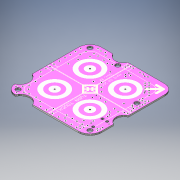
# Autodesk Inventor part: Eagle PCB rev 38
Saved by Autodesk Inventor 2016 (Build 200138000, 138)
## iProperties
Created: 2017-04-10
Part Number: Eagle PCB rev 38
Material: Generic
Document SubType Name: Modeling
Designer: Samuel Clay
Density: 1 g/cm^3
Appearance: Default
Author: Samuel Clay
Autodesk Inventor part; units mm, degrees
(part 1 of 3)
ref_plane "YZ Plane" through (0, 0, 0) normal (1, 0, 0) x (0, 1, 0)
ref_plane "XZ Plane" through (0, 0, 0) normal (0, 1, 0) x (-1, 0, 0)
ref_plane "XY Plane" through (0, 0, 0) normal (0, 0, 1) x (1, 0, 0)
sketch "PCB" plane through (0, 0, 0) normal (0, 0, 1) x (1, 0, 0)
  line L0 (18.4531, -13.3626) -> (18.4531, -8.3763)
  line L1 (17.4012, -16.4615) -> (17.5952, -16.1907)
  line L2 (4.9153, 16.5103) -> (4.4111, 16.3752)
  line L3 (13.6552, 10.6901) -> (13.633, 10.7727)
  line L4 (17.0691, 7.2094) -> (17.0086, 7.2699)
  line L5 (11.5809, 14.546) -> (11.4982, 14.5239)
  line L6 (14.6575, 2.3946) -> (14.6356, 2.4765)
  line L7 (2.2015, 12.8535) -> (2.1794, 12.9362)
  line L8 (2.1698, 12.7683) -> (2.1583, 12.8112)
  line L9 (-16.4524, -8.5544) -> (-16.6541, -8.2122)
  line L10 (2.0984, 12.8711) -> (2.0165, 12.8931)
  line L11 (-16.2848, -8.9145) -> (-16.4524, -8.5544)
  line L12 (2.1583, 12.8112) -> (2.0984, 12.8711)
  line L13 (-16.1527, -9.2892) -> (-16.2848, -8.9145)
  line L14 (2.1189, 12.9967) -> (2.0362, 13.0189)
  line L15 (-16.0575, -9.6748) -> (-16.1527, -9.2892)
  line L16 (-16, -10.0678) -> (-16.0575, -9.6748)
  line L17 (2.0362, 13.0189) -> (1.9535, 12.9967)
  line L18 (2.0165, 12.8931) -> (1.9347, 12.8711)
  line L19 (17.4509, -10.6455) -> (17.4731, -10.5628)
  line L20 (-15.9808, -10.4646) -> (-16, -10.0678)
  line L21 (-16, -10.8614) -> (-15.9808, -10.4646)
  line L22 (1.9535, 12.9967) -> (1.893, 12.9362)
  line L23 (1.9347, 12.8711) -> (1.8806, 12.8171)
  line L24 (-16.6541, -8.2122) -> (-16.8879, -7.8911)
  line L25 (2.1794, 12.9362) -> (2.1189, 12.9967)
  line L26 (1.893, 12.9362) -> (1.8709, 12.8535)
  line L27 (-18.4531, 13.3626) -> (-18.4531, -6.6988)
  line L28 (-18.0967, -6.8742) -> (-18.4531, -6.6988)
  line L29 (-17.7589, -7.0832) -> (-18.0967, -6.8742)
  line L30 (-17.4429, -7.3239) -> (-17.7589, -7.0832)
  line L31 (1.893, 12.7709) -> (1.9535, 12.7103)
  line L32 (-17.1517, -7.5941) -> (-17.4429, -7.3239)
  line L33 (-16.8879, -7.8911) -> (-17.1517, -7.5941)
  line L34 (-16.0575, -11.2544) -> (-16, -10.8614)
  line L35 (1.9535, 12.7103) -> (2.0362, 12.6882)
  line L36 (-16.1527, -11.6401) -> (-16.0575, -11.2544)
  line L37 (-16.2848, -12.0147) -> (-16.1527, -11.6401)
  line L38 (-16.4524, -12.3748) -> (-16.2848, -12.0147)
  line L39 (-16.6541, -12.717) -> (-16.4524, -12.3748)
  line L40 (-16.8879, -13.0381) -> (-16.6541, -12.717)
  line L41 (-17.1517, -13.3351) -> (-16.8879, -13.0381)
  line L42 (2.0362, 12.6882) -> (2.1189, 12.7103)
  line L43 (-17.2743, -13.4738) -> (-17.1517, -13.3351)
  line L44 (-17.5873, -13.7121) -> (-17.4429, -13.6053)
  line L45 (-18.0967, -14.055) -> (-17.7589, -13.846)
  line L46 (-17.9218, -13.9191) -> (-17.5873, -13.7121)
  line L47 (-18.4531, -14.2304) -> (-18.2747, -14.0928)
  line L48 (-18.4531, -14.2304) -> (-18.0967, -14.055)
  line L49 (-18.2747, -14.0928) -> (-17.9218, -13.9191)
  line L50 (-18.4528, -14.5799) -> (-18.4354, -14.8417)
  line L51 (-18.4354, -14.8417) -> (-18.4009, -15.1019)
  line L52 (2.1189, 12.7103) -> (2.1698, 12.7683)
  line L53 (-18.4009, -15.1019) -> (-18.3495, -15.3592)
  line L54 (-18.3495, -15.3592) -> (-18.2813, -15.6127)
  line L55 (17.3904, -10.706) -> (17.4509, -10.6455)
  line L56 (-18.2813, -15.6127) -> (-18.1967, -15.8611)
  line L57 (-18.1967, -15.8611) -> (-18.096, -16.1034)
  line L58 (-18.096, -16.1034) -> (-17.9797, -16.3387)
  line L59 (-17.9797, -16.3387) -> (-17.8483, -16.5658)
  line L60 (2.1698, 12.7683) -> (2.2015, 12.8535)
  line L61 (-17.8483, -16.5658) -> (-17.7023, -16.7839)
  line L62 (-17.7023, -16.7839) -> (-17.5423, -16.9919)
  line L63 (-17.5423, -16.9919) -> (-17.3691, -17.1891)
  line L64 (-17.3691, -17.1891) -> (-17.1833, -17.3745)
  line L65 (-17.1833, -17.3745) -> (-16.9858, -17.5473)
  line L66 (-16.9858, -17.5473) -> (-16.7775, -17.7069)
  line L67 (17.3077, -10.7282) -> (17.3904, -10.706)
  line L68 (-16.7775, -17.7069) -> (-16.5591, -17.8524)
  line L69 (-16.5591, -17.8524) -> (-16.3317, -17.9834)
  line L70 (-16.3317, -17.9834) -> (-16.0962, -18.0993)
  line L71 (-16.0962, -18.0993) -> (-15.8537, -18.1995)
  line L72 (-15.8537, -18.1995) -> (-15.6051, -18.2836)
  line L73 (-15.6051, -18.2836) -> (-15.3515, -18.3513)
  line L74 (-15.3515, -18.3513) -> (-15.0941, -18.4022)
  line L75 (-15.0941, -18.4022) -> (-14.8339, -18.4362)
  line L76 (-14.8339, -18.4362) -> (-14.572, -18.4531)
  line L77 (-14.4849, -18.4531) -> (-14.3449, -18.2747)
  line L78 (-14.572, -18.4531) -> (-14.4849, -18.4531)
  line L79 (-14.3095, -18.0967) -> (-14.4849, -18.4531)
  line L80 (-14.1712, -17.9218) -> (-14.3449, -18.2747)
  line L81 (-14.1005, -17.7589) -> (-14.3095, -18.0967)
  line L82 (-13.9642, -17.5873) -> (-14.1712, -17.9218)
  line L83 (-13.8598, -17.4429) -> (-13.9642, -17.5873)
  line L84 (17.2251, -10.706) -> (17.3077, -10.7282)
  line L85 (17.6003, 4.5815) -> (17.5782, 4.6641)
  line L86 (14.3966, -4.3715) -> (14.3361, -4.311)
  line L87 (3.3469, 15.3988) -> (3.3248, 15.4815)
  line L88 (3.3027, 15.2941) -> (3.2926, 15.3318)
  line L89 (17.5782, 4.6641) -> (17.5177, 4.7246)
  line L90 (17.5177, 4.7246) -> (17.435, 4.7468)
  line L91 (-17.0373, 12.9362) -> (-17.0978, 12.9967)
  line L92 (-17.0978, 12.9967) -> (-17.1805, 13.0189)
  line L93 (14.7784, 2.5007) -> (14.7179, 2.5612)
  line L94 (11.6108, 14.3236) -> (11.5509, 14.3835)
  line L95 (10.6455, 15.542) -> (10.5628, 15.5641)
  line L96 (10.5426, 15.3918) -> (10.4607, 15.4137)
  line L97 (-6.4904, 14.4188) -> (-6.5731, 14.3966)
  line L98 (10.5628, 15.5641) -> (10.4801, 15.542)
  line L99 (10.4607, 15.4137) -> (10.398, 15.3969)
  line L100 (-6.5731, 14.3966) -> (-6.6336, 14.3361)
  line L101 (-6.5095, 14.2575) -> (-6.5695, 14.1975)
  line L102 (10.4801, 15.542) -> (10.4196, 15.4815)
  line L103 (10.4196, 15.4815) -> (10.398, 15.3969)
  line L104 (-2.4935, 3.6943) -> (-2.5049, 3.7368)
  line L105 (10.398, 15.3969) -> (10.4196, 15.3161)
  line L106 (10.4196, 15.3161) -> (10.4801, 15.2556)
  line L107 (-6.6336, 14.3361) -> (-6.6557, 14.2534)
  line L108 (16.9042, 6.976) -> (16.9261, 7.0578)
  line L109 (10.4801, 15.2556) -> (10.5628, 15.2335)
  line L110 (-6.4077, 14.3966) -> (-6.4904, 14.4188)
  line L111 (-6.3458, 14.2575) -> (-6.4277, 14.2794)
  line L112 (-6.6557, 14.2534) -> (-6.6336, 14.1708)
  line L113 (-7.9835, 7.8903) -> (-8.0176, 7.763)
  line L114 (-2.7286, 3.7968) -> (-2.7885, 3.7368)
  line L115 (10.6455, 15.2556) -> (10.706, 15.3161)
  line L116 (10.706, 15.3161) -> (10.7282, 15.3988)
  line L117 (11.7241, 14.4634) -> (11.6636, 14.5239)
  line L118 (-6.4277, 14.2794) -> (-6.5095, 14.2575)
  line L119 (11.6636, 14.5239) -> (11.5809, 14.546)
  line L120 (-8.0176, 7.763) -> (-7.9835, 7.6358)
  line L121 (11.4982, 14.5239) -> (11.4377, 14.4634)
  line L122 (11.4377, 14.4634) -> (11.4156, 14.3807)
  line L123 (-0.8908, 17.2697) -> (-0.8082, 17.2918)
  line L124 (11.4156, 14.3807) -> (11.4377, 14.298)
  line L125 (11.4377, 14.298) -> (11.4982, 14.2375)
  line L126 (11.4982, 14.2375) -> (11.5809, 14.2154)
  line L127 (-7.6358, 7.9835) -> (-7.763, 8.0176)
  line L128 (-2.7885, 3.7368) -> (-2.8104, 3.6549)
  line L129 (-2.6467, 3.8187) -> (-2.7286, 3.7968)
  line L130 (-6.5731, 14.1102) -> (-6.4904, 14.0881)
  line L131 (11.6636, 14.2375) -> (11.7241, 14.298)
  line L132 (11.7241, 14.298) -> (11.7463, 14.3807)
  line L133 (16.7606, 7.1267) -> (16.7828, 7.044)
  line L134 (-6.5695, 14.1975) -> (-6.5887, 14.1259)
  line L135 (-0.8082, 17.2918) -> (-0.7476, 17.3523)
  line L136 (11.5509, 14.3835) -> (11.469, 14.4054)
  line L137 (11.469, 14.4054) -> (11.4156, 14.3807)
  line L138 (12.493, 13.4413) -> (12.4331, 13.5013)
  line L139 (-5.307, 13.9989) -> (-5.3291, 14.0816)
  line L140 (11.7463, 14.3807) -> (11.7241, 14.4634)
  line L141 (11.6327, 14.2417) -> (11.6108, 14.3236)
  line L142 (-7.8903, -7.5426) -> (-7.9063, -7.562)
  line L143 (16.9259, 7.2921) -> (16.8433, 7.2699)
  line L144 (-5.3291, 14.0816) -> (-5.3896, 14.1421)
  line L145 (-5.3896, 14.1421) -> (-5.4723, 14.1642)
  line L146 (4.3715, 17.5782) -> (4.311, 17.5177)
  line L147 (4.3293, 17.4083) -> (4.303, 17.3821)
  line L148 (-7.5426, -7.6358) -> (-7.6358, -7.5426)
  line L149 (-0.7255, 17.435) -> (-0.7476, 17.5177)
  line L150 (16.8442, 7.1996) -> (16.7844, 7.2157)
  line L151 (-7.763, 7.5085) -> (-7.6358, 7.5426)
  line L152 (-7.8903, 7.5426) -> (-7.763, 7.5085)
  line L153 (-0.7476, 17.5177) -> (-0.8082, 17.5782)
  line L154 (-0.7476, 17.3523) -> (-0.8004, 17.4083)
  line L155 (17.0086, 7.2699) -> (16.9259, 7.2921)
  line L156 (16.7844, 7.2157) -> (16.7606, 7.1267)
  line L157 (-0.8082, 17.5782) -> (-0.8908, 17.6003)
  line L158 (4.311, 17.5177) -> (4.2889, 17.435)
  line L159 (-0.7476, 17.3523) -> (-0.7255, 17.435)
  line L160 (-0.8004, 17.4083) -> (-0.8822, 17.4302)
  line L161 (-7.6358, -7.5426) -> (-7.763, -7.5085)
  line L162 (12.6149, 11.7908) -> (12.5544, 11.8514)
  line L163 (12.493, 11.6769) -> (12.4331, 11.7368)
  line L164 (-1.0562, 17.435) -> (-1.034, 17.3523)
  line L165 (12.6149, 13.5725) -> (12.5544, 13.633)
  line L166 (-1.034, 17.3523) -> (-0.9735, 17.2918)
  line L167 (-0.8908, 17.6003) -> (-0.9735, 17.5782)
  line L168 (12.3512, 13.5232) -> (12.3126, 13.5129)
  line L169 (-0.9735, 17.5782) -> (-1.034, 17.5177)
  line L170 (-1.034, 17.5177) -> (-1.0562, 17.435)
  line L171 (12.515, 13.3595) -> (12.493, 13.4413)
  line L172 (13.633, 12.5544) -> (13.5725, 12.6149)
  line L173 (-0.8822, 17.4302) -> (-0.9641, 17.4083)
  line L174 (13.5725, 12.6149) -> (13.4899, 12.6371)
  line L175 (12.4331, 13.5013) -> (12.3512, 13.5232)
  line L176 (12.5082, 13.3343) -> (12.515, 13.3595)
  line L177 (12.6371, 13.4899) -> (12.6149, 13.5725)
  line L178 (-7.8903, 7.9835) -> (-7.9835, 7.8903)
  line L179 (12.5544, 13.633) -> (12.4718, 13.6552)
  line L180 (16.9259, 6.9614) -> (17.0086, 6.9835)
  line L181 (12.4718, 13.6552) -> (12.3891, 13.633)
  line L182 (12.3891, 13.633) -> (12.3286, 13.5725)
  line L183 (12.3064, 13.4899) -> (12.3286, 13.4072)
  line L184 (12.3286, 13.4072) -> (12.3891, 13.3467)
  line L185 (16.7828, 7.044) -> (16.8433, 6.9835)
  line L186 (12.3891, 13.3467) -> (12.4718, 13.3245)
  line L187 (12.5544, 13.3467) -> (12.6149, 13.4072)
  line L188 (12.6149, 13.4072) -> (12.6371, 13.4899)
  line L189 (4.4542, 17.6003) -> (4.3715, 17.5782)
  line L190 (4.4111, 17.4302) -> (4.3293, 17.4083)
  line L191 (12.599, 2.889) -> (12.6817, 2.9111)
  line L192 (13.6552, 12.4718) -> (13.633, 12.5544)
  line L193 (13.3467, 12.3891) -> (13.4072, 12.3286)
  line L194 (13.4899, 12.6371) -> (13.4072, 12.6149)
  line L195 (13.4072, 12.6149) -> (13.3467, 12.5544)
  line L196 (13.3245, 12.4718) -> (13.3467, 12.3891)
  line L197 (13.4072, 12.3286) -> (13.4899, 12.3064)
  line L198 (-7.6358, 7.5426) -> (-7.5426, 7.6358)
  line L199 (13.5725, 12.3286) -> (13.633, 12.3891)
  line L200 (16.9042, 7.1397) -> (16.8442, 7.1996)
  line L201 (13.633, 12.3891) -> (13.6552, 12.4718)
  line L202 (16.8433, 7.2699) -> (16.7844, 7.2157)
  line L203 (6.8881, 14.8071) -> (6.9103, 14.8897)
  line L204 (-0.9641, 17.4083) -> (-1.034, 17.3523)
  line L205 (12.515, 11.595) -> (12.493, 11.6769)
  line L206 (14.4496, 11.4848) -> (14.3677, 11.5067)
  line L207 (13.5232, 12.3512) -> (13.5013, 12.4331)
  line L208 (13.5013, 12.4331) -> (13.4413, 12.493)
  line L209 (13.4413, 12.493) -> (13.3595, 12.515)
  line L210 (13.3595, 12.515) -> (13.3343, 12.5082)
  line L211 (14.5095, 11.4248) -> (14.4496, 11.4848)
  line L212 (13.5129, 12.3126) -> (13.5232, 12.3512)
  line L213 (6.5796, 14.8897) -> (6.6017, 14.8071)
  line L214 (6.9103, 14.8897) -> (6.8881, 14.9724)
  line L215 (6.8422, 14.7505) -> (6.8215, 14.8277)
  line L216 (-7.9063, -7.562) -> (-7.9401, -7.688)
  line L217 (6.6017, 14.8071) -> (6.6623, 14.7466)
  line L218 (6.7449, 15.0551) -> (6.6623, 15.0329)
  line L219 (6.8422, 14.7505) -> (6.8881, 14.8071)
  line L220 (-7.9835, -7.6358) -> (-8.0176, -7.763)
  line L221 (-7.688, -7.9401) -> (-7.562, -7.9063)
  line L222 (6.6623, 15.0329) -> (6.6017, 14.9724)
  line L223 (-7.8903, -7.9835) -> (-7.763, -8.0176)
  line L224 (6.6017, 14.9724) -> (6.5796, 14.8897)
  line L225 (-7.9063, -7.814) -> (-7.814, -7.9063)
  line L226 (6.6623, 14.7466) -> (6.7449, 14.7244)
  line L227 (6.7449, 14.7244) -> (6.8422, 14.7505)
  line L228 (-7.763, -8.0176) -> (-7.6358, -7.9835)
  line L229 (4.5369, 17.5782) -> (4.4542, 17.6003)
  line L230 (4.493, 17.4083) -> (4.4111, 17.4302)
  line L231 (6.8881, 14.9724) -> (6.8276, 15.0329)
  line L232 (6.8215, 14.8277) -> (6.7616, 14.8876)
  line L233 (14.6511, 11.5363) -> (14.5906, 11.5968)
  line L234 (14.5315, 11.3429) -> (14.5095, 11.4248)
  line L235 (14.5162, 11.2861) -> (14.5315, 11.3429)
  line L236 (14.6733, 11.4536) -> (14.6511, 11.5363)
  line L237 (14.5906, 11.5968) -> (14.508, 11.619)
  line L238 (14.4253, 11.5968) -> (14.359, 11.5435)
  line L239 (14.508, 11.619) -> (14.4253, 11.5968)
  line L240 (14.3426, 11.4536) -> (14.3648, 11.371)
  line L241 (14.3648, 11.371) -> (14.4253, 11.3105)
  line L242 (14.4253, 11.3105) -> (14.5162, 11.2861)
  line L243 (14.5162, 11.2861) -> (14.5906, 11.3105)
  line L244 (14.5906, 11.3105) -> (14.6511, 11.371)
  line L245 (14.6511, 11.371) -> (14.6733, 11.4536)
  line L246 (4.5974, 17.3523) -> (4.6195, 17.435)
  line L247 (8.4153, 17.5177) -> (8.3548, 17.5782)
  line L248 (8.3548, 17.5782) -> (8.2721, 17.6003)
  line L249 (7.1426, 15.9905) -> (7.0821, 16.051)
  line L250 (8.1289, 17.3523) -> (8.1894, 17.2918)
  line L251 (8.2721, 17.6003) -> (8.1894, 17.5782)
  line L252 (8.1894, 17.5782) -> (8.1289, 17.5177)
  line L253 (-7.814, -7.9063) -> (-7.688, -7.9401)
  line L254 (8.1289, 17.5177) -> (8.1067, 17.435)
  line L255 (8.4374, 17.435) -> (8.4153, 17.5177)
  line L256 (8.1894, 17.2918) -> (8.2721, 17.2697)
  line L257 (8.2721, 17.2697) -> (8.3548, 17.2918)
  line L258 (8.3548, 17.2918) -> (8.4153, 17.3523)
  line L259 (8.4153, 17.3523) -> (8.4374, 17.435)
  line L260 (6.8276, 15.0329) -> (6.7449, 15.0551)
  line L261 (5.4564, 17.5177) -> (5.4342, 17.435)
  line L262 (5.6822, 17.5782) -> (5.5996, 17.6003)
  line L263 (8.3548, 17.2918) -> (8.3339, 17.3484)
  line L264 (8.3339, 17.3484) -> (8.274, 17.4083)
  line L265 (8.274, 17.4083) -> (8.1921, 17.4302)
  line L266 (8.1921, 17.4302) -> (8.1137, 17.4092)
  line L267 (6.6797, 14.9096) -> (6.5796, 14.8897)
  line L268 (5.5169, 17.5782) -> (5.4564, 17.5177)
  line L269 (5.5996, 17.6003) -> (5.5169, 17.5782)
  line L270 (5.7428, 17.5177) -> (5.6822, 17.5782)
  line L271 (5.4564, 17.3523) -> (5.5169, 17.2918)
  line L272 (-7.763, -7.5085) -> (-7.8903, -7.5426)
  line L273 (5.5169, 17.2918) -> (5.5996, 17.2697)
  line L274 (-8.0176, -7.763) -> (-7.9835, -7.8903)
  line L275 (-7.9401, -7.688) -> (-7.9063, -7.814)
  line L276 (6.7616, 14.8876) -> (6.6797, 14.9096)
  line L277 (-7.5426, -7.8903) -> (-7.5085, -7.763)
  line L278 (5.7649, 17.435) -> (5.7428, 17.5177)
  line L279 (4.3715, 17.2918) -> (4.4542, 17.2697)
  line L280 (4.4542, 17.2697) -> (4.5369, 17.2918)
  line L281 (5.5996, 17.2697) -> (5.6822, 17.2918)
  line L282 (5.7428, 17.3523) -> (5.7649, 17.435)
  line L283 (5.6981, 17.3077) -> (5.6872, 17.3484)
  line L284 (4.6195, 17.435) -> (4.5974, 17.5177)
  line L285 (4.5615, 17.3164) -> (4.553, 17.3484)
  line L286 (-7.9835, -7.8903) -> (-7.8903, -7.9835)
  line L287 (5.6872, 17.3484) -> (5.6273, 17.4083)
  line L288 (5.6273, 17.4083) -> (5.5454, 17.4302)
  line L289 (5.5454, 17.4302) -> (5.4636, 17.4083)
  line L290 (5.4636, 17.4083) -> (5.4461, 17.3908)
  line L291 (-7.5085, -7.763) -> (-7.5426, -7.6358)
  line L292 (4.5974, 17.5177) -> (4.5369, 17.5782)
  line L293 (4.553, 17.3484) -> (4.493, 17.4083)
  line L294 (-7.562, -7.9063) -> (-7.5426, -7.8903)
  line L295 (4.311, 17.3523) -> (4.3715, 17.2918)
  line L296 (6.9103, 17.435) -> (6.8881, 17.5177)
  line L297 (6.8881, 17.5177) -> (6.8276, 17.5782)
  line L298 (6.8276, 17.5782) -> (6.7449, 17.6003)
  line L299 (6.6017, 17.3523) -> (6.6623, 17.2918)
  line L300 (6.7449, 17.6003) -> (6.6623, 17.5782)
  line L301 (6.6623, 17.5782) -> (6.6017, 17.5177)
  line L302 (6.6017, 17.5177) -> (6.5796, 17.435)
  line L303 (6.8361, 17.2941) -> (6.8215, 17.3484)
  line L304 (6.6623, 17.2918) -> (6.7449, 17.2697)
  line L305 (6.7449, 17.2697) -> (6.8361, 17.2941)
  line L306 (6.8361, 17.2941) -> (6.8881, 17.3523)
  line L307 (6.8881, 17.3523) -> (6.9103, 17.435)
  line L308 (3.0989, 15.2556) -> (3.1816, 15.2335)
  line L309 (3.0689, 15.3918) -> (3.0289, 15.3517)
  line L310 (17.435, 7.8522) -> (17.5177, 7.8744)
  line L311 (6.8215, 17.3484) -> (6.7616, 17.4083)
  line L312 (12.5544, 11.8514) -> (12.4718, 11.8735)
  line L313 (6.7616, 17.4083) -> (6.6797, 17.4302)
  line L314 (6.6797, 17.4302) -> (6.5979, 17.4083)
  line L315 (12.3286, 11.6255) -> (12.3891, 11.565)
  line L316 (12.4718, 11.8735) -> (12.3891, 11.8514)
  line L317 (12.3891, 11.8514) -> (12.3286, 11.7908)
  line L318 (12.3064, 11.7082) -> (12.3286, 11.6255)
  line L319 (12.3891, 11.565) -> (12.4718, 11.5428)
  line L320 (12.5544, 11.565) -> (12.6149, 11.6255)
  line L321 (3.2642, 15.542) -> (3.1816, 15.5641)
  line L322 (12.6149, 11.6255) -> (12.6371, 11.7082)
  line L323 (3.0384, 15.3161) -> (3.0989, 15.2556)
  line L324 (3.1816, 15.5641) -> (3.0989, 15.542)
  line L325 (3.0989, 15.542) -> (3.0384, 15.4815)
  line L326 (17.6003, 8.0176) -> (17.5782, 8.1002)
  line L327 (17.5782, 8.1002) -> (17.5177, 8.1607)
  line L328 (17.5177, 8.1607) -> (17.435, 8.1829)
  line L329 (17.2918, 7.9349) -> (17.3523, 7.8744)
  line L330 (12.6371, 11.7082) -> (12.6149, 11.7908)
  line L331 (3.0384, 15.4815) -> (3.0162, 15.3988)
  line L332 (17.435, 8.1829) -> (17.3523, 8.1607)
  line L333 (17.3523, 8.1607) -> (17.2918, 8.1002)
  line L334 (17.2918, 8.1002) -> (17.2697, 8.0176)
  line L335 (17.2697, 8.0176) -> (17.2918, 7.9349)
  line L336 (17.5177, 7.8744) -> (17.5782, 7.9349)
  line L337 (17.5782, 7.9349) -> (17.6003, 8.0176)
  line L338 (3.1508, 15.4137) -> (3.0689, 15.3918)
  line L339 (3.2327, 15.3918) -> (3.1508, 15.4137)
  line L340 (3.2926, 15.3318) -> (3.2327, 15.3918)
  line L341 (2.1635, 17.0913) -> (2.0808, 17.0691)
  line L342 (2.1426, 16.9261) -> (2.0607, 16.9042)
  line L343 (17.3523, 0.2386) -> (17.435, 0.2164)
  line L344 (17.4302, 5.9235) -> (17.4083, 6.0054)
  line L345 (15.3161, 10.706) -> (15.2556, 10.6455)
  line L346 (17.4083, 6.0054) -> (17.3484, 6.0653)
  line L347 (17.3484, 6.0653) -> (17.2959, 6.0794)
  line L348 (17.5782, 6.064) -> (17.5177, 6.1245)
  line L349 (13.3595, 10.7505) -> (13.3392, 10.7451)
  line L350 (17.3937, 5.8271) -> (17.4083, 5.8417)
  line L351 (17.4083, 5.8417) -> (17.4302, 5.9235)
  line L352 (17.6003, 5.9813) -> (17.5782, 6.064)
  line L353 (15.2335, 10.5628) -> (15.2556, 10.4801)
  line L354 (17.5177, 6.1245) -> (17.435, 6.1467)
  line L355 (15.3161, 10.4196) -> (15.3988, 10.3975)
  line L356 (17.435, 6.1467) -> (17.3523, 6.1245)
  line L357 (15.3988, 10.3975) -> (15.4815, 10.4196)
  line L358 (17.3523, 6.1245) -> (17.2959, 6.0794)
  line L359 (15.4815, 10.4196) -> (15.542, 10.4801)
  line L360 (15.542, 10.4801) -> (15.5641, 10.5628)
  line L361 (17.2959, 6.0794) -> (17.2697, 5.9813)
  line L362 (13.5232, 10.5868) -> (13.5013, 10.6686)
  line L363 (17.2697, 5.9813) -> (17.2918, 5.8987)
  line L364 (17.2918, 5.8987) -> (17.3523, 5.8382)
  line L365 (17.435, 5.816) -> (17.5177, 5.8382)
  line L366 (17.5177, 5.8382) -> (17.5782, 5.8987)
  line L367 (17.5782, 5.8987) -> (17.6003, 5.9813)
  line L368 (14.2915, 3.6906) -> (14.2694, 3.7733)
  line L369 (17.6003, 0.3818) -> (17.5782, 0.4645)
  line L370 (2.3067, 16.8433) -> (2.3288, 16.9259)
  line L371 (17.5782, 0.4645) -> (17.5177, 0.525)
  line L372 (15.5641, 10.5628) -> (15.542, 10.6455)
  line L373 (17.5177, 0.525) -> (17.435, 0.5471)
  line L374 (17.2918, 0.2991) -> (17.3523, 0.2386)
  line L375 (17.435, 0.5471) -> (17.3523, 0.525)
  line L376 (15.542, 10.6455) -> (15.4815, 10.706)
  line L377 (17.3523, 0.525) -> (17.2918, 0.4645)
  line L378 (2.3067, 17.0086) -> (2.2461, 17.0691)
  line L379 (2.2844, 16.8442) -> (2.2244, 16.9042)
  line L380 (17.2918, 0.4645) -> (17.2697, 0.3818)
  line L381 (17.2697, 0.3818) -> (17.2918, 0.2991)
  line L382 (17.435, 0.2164) -> (17.5177, 0.2386)
  line L383 (17.5177, 0.2386) -> (17.5782, 0.2991)
  line L384 (17.5782, 0.2991) -> (17.6003, 0.3818)
  line L385 (14.2794, -4.4111) -> (14.2575, -4.3293)
  line L386 (1.6186, 3.4114) -> (1.6542, 3.447)
  line L387 (17.4302, 0.3781) -> (17.4083, 0.46)
  line L388 (17.4083, 0.46) -> (17.3523, 0.525)
  line L389 (17.3523, 0.2386) -> (17.4083, 0.2962)
  line L390 (17.4083, 0.2962) -> (17.4302, 0.3781)
  line L391 (2.2461, 17.0691) -> (2.1635, 17.0913)
  line L392 (2.2244, 16.9042) -> (2.1426, 16.9261)
  line L393 (2.0808, 17.0691) -> (2.0203, 17.0086)
  line L394 (2.0607, 16.9042) -> (2.01, 16.8535)
  line L395 (2.0808, 16.7828) -> (2.1635, 16.7606)
  line L396 (2.1635, 16.7606) -> (2.2461, 16.7828)
  line L397 (13.3467, 10.6074) -> (13.4072, 10.5469)
  line L398 (14.4188, -4.4542) -> (14.3966, -4.3715)
  line L399 (2.0203, 17.0086) -> (1.9981, 16.9259)
  line L400 (14.2575, -4.3293) -> (14.2247, -4.2965)
  line L401 (14.3361, -4.311) -> (14.2542, -4.2864)
  line L402 (14.1414, -4.568) -> (14.1975, -4.553)
  line L403 (14.1975, -4.553) -> (14.2575, -4.493)
  line L404 (14.2575, -4.493) -> (14.2794, -4.4111)
  line L405 (14.1708, -4.311) -> (14.1102, -4.3715)
  line L406 (1.9981, 16.9259) -> (2.01, 16.8535)
  line L407 (14.1102, -4.3715) -> (14.0881, -4.4542)
  line L408 (14.0881, -4.4542) -> (14.1102, -4.5369)
  line L409 (2.01, 16.8535) -> (2.0808, 16.7828)
  line L410 (14.1708, -4.5974) -> (14.2534, -4.6195)
  line L411 (14.2534, -4.6195) -> (14.3361, -4.5974)
  line L412 (14.3361, -4.5974) -> (14.3966, -4.5369)
  line L413 (14.3966, -4.5369) -> (14.4188, -4.4542)
  line L414 (13.633, 10.6074) -> (13.6552, 10.6901)
  line L415 (13.5055, 10.5205) -> (13.5232, 10.5868)
  line L416 (17.4731, -10.5628) -> (17.4509, -10.4801)
  line L417 (17.4509, -10.4801) -> (17.3904, -10.4196)
  line L418 (17.3904, -10.4196) -> (17.3077, -10.3975)
  line L419 (17.1645, -10.6455) -> (17.2251, -10.706)
  line L420 (2.3288, 16.9259) -> (2.3067, 17.0086)
  line L421 (13.3245, 10.6901) -> (13.3467, 10.6074)
  line L422 (17.2251, -10.4196) -> (17.1645, -10.4801)
  line L423 (17.1645, -10.4801) -> (17.1424, -10.5628)
  line L424 (13.4899, 10.8554) -> (13.4072, 10.8333)
  line L425 (13.4072, 10.8333) -> (13.341, 10.7798)
  line L426 (15.5839, -7.0736) -> (15.6438, -7.0137)
  line L427 (17.3042, -10.4607) -> (17.2886, -10.4026)
  line L428 (13.5725, 10.5469) -> (13.633, 10.6074)
  line L429 (13.5055, 10.5205) -> (13.5725, 10.5469)
  line L430 (13.5725, 10.8333) -> (13.4899, 10.8554)
  line L431 (13.4413, 10.7286) -> (13.3595, 10.7505)
  line L432 (17.1577, -10.6198) -> (17.2223, -10.6025)
  line L433 (17.2223, -10.6025) -> (17.2823, -10.5426)
  line L434 (17.2823, -10.5426) -> (17.3042, -10.4607)
  line L435 (13.633, 10.7727) -> (13.5725, 10.8333)
  line L436 (13.5013, 10.6686) -> (13.4413, 10.7286)
  line L437 (15.736, -6.8563) -> (15.6584, -6.8225)
  line L438 (1.6098, 3.7065) -> (1.5272, 3.7287)
  line L439 (1.5943, 3.6707) -> (1.5124, 3.6927)
  line L440 (13.4072, 10.5469) -> (13.5055, 10.5205)
  line L441 (15.8187, -6.9995) -> (15.7965, -6.9168)
  line L442 (15.6658, -6.9318) -> (15.6438, -6.8499)
  line L443 (15.5129, -7.0926) -> (15.5839, -7.0736)
  line L444 (15.6438, -7.0137) -> (15.6658, -6.9318)
  line L445 (12.5163, 3.1975) -> (12.4558, 3.137)
  line L446 (15.7965, -6.9168) -> (15.736, -6.8563)
  line L447 (15.6584, -6.8225) -> (15.5706, -6.8563)
  line L448 (12.599, 3.2196) -> (12.5163, 3.1975)
  line L449 (15.5706, -6.8563) -> (15.5101, -6.9168)
  line L450 (17.435, -0.5982) -> (17.3523, -0.6204)
  line L451 (12.5723, 2.8961) -> (12.619, 2.9429)
  line L452 (15.5101, -6.9168) -> (15.488, -6.9995)
  line L453 (12.619, 2.9429) -> (12.641, 3.0248)
  line L454 (15.488, -6.9995) -> (15.5129, -7.0926)
  line L455 (17.4083, -0.6743) -> (17.3523, -0.6204)
  line L456 (15.5129, -7.0926) -> (15.5706, -7.1426)
  line L457 (17.2918, -0.6809) -> (17.2697, -0.7636)
  line L458 (15.5706, -7.1426) -> (15.6533, -7.1648)
  line L459 (17.4302, -0.7562) -> (17.4083, -0.6743)
  line L460 (15.6533, -7.1648) -> (15.736, -7.1426)
  line L461 (15.736, -7.1426) -> (15.7965, -7.0821)
  line L462 (15.7965, -7.0821) -> (15.8187, -6.9995)
  line L463 (12.4558, 2.9716) -> (12.5163, 2.9111)
  line L464 (15.997, -0.6363) -> (16.0192, -0.719)
  line L465 (14.546, -10.8173) -> (14.5239, -10.7347)
  line L466 (14.5239, -10.7347) -> (14.4634, -10.6741)
  line L467 (14.4634, -10.6741) -> (14.3807, -10.652)
  line L468 (14.2375, -10.9) -> (14.298, -10.9605)
  line L469 (14.3807, -10.652) -> (14.298, -10.6741)
  line L470 (14.298, -10.6741) -> (14.2375, -10.7347)
  line L471 (12.7422, 3.137) -> (12.6817, 3.1975)
  line L472 (12.619, 3.1067) -> (12.5591, 3.1666)
  line L473 (14.2375, -10.7347) -> (14.2154, -10.8173)
  line L474 (12.641, 3.0248) -> (12.619, 3.1067)
  line L475 (12.7644, 3.0543) -> (12.7422, 3.137)
  line L476 (12.3445, -12.1791) -> (12.2618, -12.2013)
  line L477 (14.298, -10.9605) -> (14.3807, -10.9827)
  line L478 (14.3807, -10.9827) -> (14.4634, -10.9605)
  line L479 (14.4634, -10.9605) -> (14.5239, -10.9)
  line L480 (14.5239, -10.9) -> (14.546, -10.8173)
  line L481 (17.6003, -0.7636) -> (17.5782, -0.6809)
  line L482 (12.5591, 3.1666) -> (12.5163, 3.1975)
  line L483 (14.4054, -10.7128) -> (14.3807, -10.652)
  line L484 (17.2918, -0.8462) -> (17.3523, -0.9068)
  line L485 (14.2417, -10.8765) -> (14.3236, -10.8546)
  line L486 (14.3236, -10.8546) -> (14.3835, -10.7947)
  line L487 (14.3835, -10.7947) -> (14.4054, -10.7128)
  line L488 (-2.1189, 12.9967) -> (-2.1794, 12.9362)
  line L489 (17.0913, -12.09) -> (17.0691, -12.0073)
  line L490 (16.9261, -11.9731) -> (16.914, -11.9278)
  line L491 (17.5782, -0.6809) -> (17.5177, -0.6204)
  line L492 (17.3523, -0.6204) -> (17.2918, -0.6809)
  line L493 (-2.0362, 12.6882) -> (-1.9535, 12.7103)
  line L494 (16.3277, -0.6363) -> (16.3056, -0.5536)
  line L495 (17.2697, -0.7636) -> (17.2918, -0.8462)
  line L496 (17.3523, -0.9068) -> (17.4083, -0.8381)
  line L497 (-1.893, 12.9362) -> (-1.9535, 12.9967)
  line L498 (17.4083, -0.8381) -> (17.4302, -0.7562)
  line L499 (17.3523, -0.9068) -> (17.435, -0.9289)
  line L500 (17.5177, -0.6204) -> (17.435, -0.5982)
  line L501 (-2.2015, 12.8535) -> (-2.1794, 12.7709)
  line L502 (16.7724, -12.1342) -> (16.8442, -12.1149)
  line L503 (16.8442, -12.1149) -> (16.9042, -12.055)
  line L504 (16.9042, -12.055) -> (16.9261, -11.9731)
  line L505 (17.0691, -12.0073) -> (17.0086, -11.9468)
  line L506 (17.0086, -11.9468) -> (16.914, -11.9278)
  line L507 (16.245, -0.4931) -> (16.1624, -0.471)
  line L508 (-1.9535, 12.7103) -> (-1.893, 12.7709)
  line L509 (16.914, -11.9278) -> (16.8433, -11.9468)
  line L510 (-1.8709, 12.8535) -> (-1.893, 12.9362)
  line L511 (-2.0165, 12.8931) -> (-2.0984, 12.8711)
  line L512 (16.8433, -11.9468) -> (16.7828, -12.0073)
  line L513 (16.0192, -0.719) -> (16.0797, -0.7795)
  line L514 (16.7828, -12.0073) -> (16.7606, -12.09)
  line L515 (-2.1583, 12.8112) -> (-2.1794, 12.7709)
  line L516 (16.1624, -0.471) -> (16.0797, -0.4931)
  line L517 (16.7828, -12.1726) -> (16.8433, -12.2332)
  line L518 (16.0797, -0.4931) -> (16.0192, -0.5536)
  line L519 (16.8433, -12.2332) -> (16.9259, -12.2553)
  line L520 (12.2618, -12.2013) -> (12.2013, -12.2618)
  line L521 (16.9259, -12.2553) -> (17.0086, -12.2332)
  line L522 (17.0086, -12.2332) -> (17.0691, -12.1726)
  line L523 (16.0192, -0.5536) -> (15.997, -0.6363)
  line L524 (17.0691, -12.1726) -> (17.0913, -12.09)
  line L525 (-2.0362, 13.0189) -> (-2.1189, 12.9967)
  line L526 (17.3458, -13.6171) -> (17.3237, -13.5344)
  line L527 (17.3237, -13.5344) -> (17.2631, -13.4739)
  line L528 (17.2631, -13.4739) -> (17.1805, -13.4518)
  line L529 (17.0373, -13.6998) -> (17.0978, -13.7603)
  line L530 (17.1805, -13.4518) -> (17.0978, -13.4739)
  line L531 (-1.9535, 12.9967) -> (-2.0362, 13.0189)
  line L532 (17.0978, -13.4739) -> (17.0373, -13.5344)
  line L533 (17.0373, -13.5344) -> (17.0151, -13.6171)
  line L534 (-2.1794, 12.9362) -> (-2.2015, 12.8535)
  line L535 (-2.0984, 12.8711) -> (-2.1583, 12.8112)
  line L536 (17.0978, -13.7603) -> (17.1805, -13.7825)
  line L537 (-2.1189, 12.7103) -> (-2.0362, 12.6882)
  line L538 (17.1805, -13.7825) -> (17.2631, -13.7603)
  line L539 (17.2631, -13.7603) -> (17.3237, -13.6998)
  line L540 (-2.1794, 12.7709) -> (-2.1189, 12.7103)
  line L541 (17.3237, -13.6998) -> (17.3458, -13.6171)
  line L542 (-1.8806, 12.8171) -> (-1.9347, 12.8711)
  line L543 (10.9892, -15.2556) -> (10.9287, -15.3161)
  line L544 (10.9287, -15.3161) -> (10.9065, -15.3988)
  line L545 (10.9065, -15.3988) -> (10.9287, -15.4815)
  line L546 (10.9287, -15.4815) -> (10.9892, -15.542)
  line L547 (10.9892, -15.542) -> (11.0719, -15.5641)
  line L548 (11.0719, -15.5641) -> (11.1545, -15.542)
  line L549 (11.1545, -15.542) -> (11.215, -15.4815)
  line L550 (11.215, -15.4815) -> (11.2372, -15.3988)
  line L551 (-1.9347, 12.8711) -> (-2.0165, 12.8931)
  line L552 (11.215, -15.3161) -> (11.1651, -15.2479)
  line L553 (12.3445, -12.5098) -> (12.4272, -12.4877)
  line L554 (13.2799, -17.5782) -> (13.3626, -17.6003)
  line L555 (13.3626, -17.6003) -> (13.4453, -17.5782)
  line L556 (-2.418, 14.5971) -> (-2.3353, 14.6193)
  line L557 (10.9065, -15.3988) -> (10.9648, -15.4137)
  line L558 (12.5098, -12.3445) -> (12.4877, -12.2618)
  line L559 (12.3889, -12.2252) -> (12.3791, -12.1884)
  line L560 (10.9648, -15.4137) -> (11.0467, -15.3918)
  line L561 (11.0467, -15.3918) -> (11.1067, -15.3318)
  line L562 (11.1067, -15.3318) -> (11.1286, -15.25)
  line L563 (12.2013, -12.4272) -> (12.2618, -12.4877)
  line L564 (11.2372, -15.3988) -> (11.215, -15.3161)
  line L565 (12.1884, -12.3791) -> (12.2252, -12.3889)
  line L566 (11.0719, -15.2335) -> (10.9892, -15.2556)
  line L567 (12.2013, -12.2618) -> (12.1791, -12.3445)
  line L568 (-2.5007, 14.6193) -> (-2.418, 14.5971)
  line L569 (13.5279, -17.435) -> (13.5058, -17.3523)
  line L570 (13.5058, -17.3523) -> (13.4453, -17.2918)
  line L571 (12.4877, -12.2618) -> (12.4272, -12.2013)
  line L572 (13.2194, -17.5177) -> (13.2799, -17.5782)
  line L573 (13.3626, -17.2697) -> (13.2799, -17.2918)
  line L574 (12.4272, -12.4877) -> (12.4877, -12.4272)
  line L575 (13.2799, -17.2918) -> (13.2194, -17.3523)
  line L576 (13.2194, -17.3523) -> (13.1972, -17.435)
  line L577 (13.1972, -17.435) -> (13.2194, -17.5177)
  line L578 (13.4453, -17.5782) -> (13.5058, -17.5177)
  line L579 (13.5058, -17.5177) -> (13.5279, -17.435)
  line L580 (-2.5833, 14.7625) -> (-2.5612, 14.6798)
  line L581 (-2.5612, 14.6798) -> (-2.5007, 14.6193)
  line L582 (13.1972, -17.435) -> (13.2334, -17.4302)
  line L583 (14.0435, -7.8744) -> (13.983, -7.9349)
  line L584 (13.2334, -17.4302) -> (13.3153, -17.4083)
  line L585 (13.3153, -17.4083) -> (13.3752, -17.3484)
  line L586 (13.3752, -17.3484) -> (13.3941, -17.2781)
  line L587 (13.983, -8.1002) -> (14.0435, -8.1607)
  line L588 (14.1262, -7.8522) -> (14.0435, -7.8744)
  line L589 (11.2372, -17.435) -> (11.215, -17.3523)
  line L590 (11.215, -17.3523) -> (11.1696, -17.282)
  line L591 (13.983, -7.9349) -> (13.9608, -8.0176)
  line L592 (13.9608, -8.0176) -> (13.983, -8.1002)
  line L593 (12.4877, -12.4272) -> (12.5098, -12.3445)
  line L594 (12.367, -12.307) -> (12.3889, -12.2252)
  line L595 (14.0435, -8.1607) -> (14.1262, -8.1829)
  line L596 (14.1262, -8.1829) -> (14.2088, -8.1607)
  line L597 (14.2088, -8.1607) -> (14.2694, -8.1002)
  line L598 (14.2694, -8.1002) -> (14.2915, -8.0176)
  line L599 (12.307, -12.367) -> (12.367, -12.307)
  line L600 (-2.5612, 14.8452) -> (-2.5833, 14.7625)
  line L601 (-2.5364, 14.7017) -> (-2.5612, 14.6798)
  line L602 (12.2252, -12.3889) -> (12.307, -12.367)
  line L603 (8.7811, -17.6003) -> (8.8638, -17.5782)
  line L604 (8.8638, -17.5782) -> (8.9243, -17.5177)
  line L605 (10.9116, -17.416) -> (10.9648, -17.4302)
  line L606 (10.9648, -17.4302) -> (11.0467, -17.4083)
  line L607 (11.0467, -17.4083) -> (11.1067, -17.3484)
  line L608 (11.1067, -17.3484) -> (11.124, -17.2836)
  line L609 (12.2618, -12.4877) -> (12.3445, -12.5098)
  line L610 (11.0719, -17.2697) -> (10.9892, -17.2918)
  line L611 (10.9892, -17.2918) -> (10.9287, -17.3523)
  line L612 (10.9065, -17.435) -> (10.9287, -17.5177)
  line L613 (10.9287, -17.5177) -> (10.9892, -17.5782)
  line L614 (10.9892, -17.5782) -> (11.0719, -17.6003)
  line L615 (11.0719, -17.6003) -> (11.1545, -17.5782)
  line L616 (11.1545, -17.5782) -> (11.215, -17.5177)
  line L617 (11.215, -17.5177) -> (11.2372, -17.435)
  line L618 (-2.5007, 14.9057) -> (-2.5612, 14.8452)
  line L619 (-2.4765, 14.7616) -> (-2.5364, 14.7017)
  line L620 (8.9465, -17.435) -> (8.9243, -17.3523)
  line L621 (8.9243, -17.3523) -> (8.8638, -17.2918)
  line L622 (8.8638, -17.2918) -> (8.7811, -17.2697)
  line L623 (8.6379, -17.5177) -> (8.6985, -17.5782)
  line L624 (8.7811, -17.2697) -> (8.6985, -17.2918)
  line L625 (8.6985, -17.2918) -> (8.6379, -17.3523)
  line L626 (8.6158, -17.435) -> (8.6379, -17.5177)
  line L627 (8.6985, -17.5782) -> (8.7811, -17.6003)
  line L628 (8.9243, -17.5177) -> (8.9465, -17.435)
  line L629 (-13.4899, 16.8368) -> (-13.5725, 16.8146)
  line L630 (-13.3595, 16.674) -> (-13.4413, 16.6521)
  line L631 (-2.418, 14.9278) -> (-2.5007, 14.9057)
  line L632 (-2.3946, 14.7835) -> (-2.4765, 14.7616)
  line L633 (3.8625, -17.5782) -> (3.9451, -17.6003)
  line L634 (3.9451, -17.6003) -> (4.0278, -17.5782)
  line L635 (-2.2748, 14.8452) -> (-2.3353, 14.9057)
  line L636 (-2.2655, 14.7144) -> (-2.3128, 14.7616)
  line L637 (8.6224, -17.4104) -> (8.6963, -17.4302)
  line L638 (8.4884, -13.8794) -> (8.5702, -13.9013)
  line L639 (8.6963, -17.4302) -> (8.7781, -17.4083)
  line L640 (8.7781, -17.4083) -> (8.8381, -17.3484)
  line L641 (8.8381, -17.3484) -> (8.8638, -17.2918)
  line L642 (-2.2527, 14.7625) -> (-2.2748, 14.8452)
  line L643 (8.5702, -13.9013) -> (8.6521, -13.8794)
  line L644 (8.6521, -13.8794) -> (8.712, -13.8194)
  line L645 (8.712, -13.8194) -> (8.734, -13.7376)
  line L646 (-2.3353, 14.9057) -> (-2.418, 14.9278)
  line L647 (-2.3128, 14.7616) -> (-2.3946, 14.7835)
  line L648 (4.1105, -17.435) -> (4.0883, -17.3523)
  line L649 (4.0278, -17.2918) -> (3.9451, -17.2697)
  line L650 (3.802, -17.5177) -> (3.8625, -17.5782)
  line L651 (3.9451, -17.2697) -> (3.8625, -17.2918)
  line L652 (3.8625, -17.2918) -> (3.802, -17.3523)
  line L653 (3.7798, -17.435) -> (3.802, -17.5177)
  line L654 (4.0278, -17.5782) -> (4.0883, -17.5177)
  line L655 (4.0883, -17.5177) -> (4.1105, -17.435)
  line L656 (-13.5725, 16.8146) -> (-13.633, 16.7541)
  line L657 (-13.4413, 16.6521) -> (-13.5013, 16.5922)
  line L658 (1.5717, -17.5782) -> (1.6544, -17.6003)
  line L659 (1.6544, -17.6003) -> (1.7371, -17.5782)
  line L660 (3.795, -17.3782) -> (3.8251, -17.4083)
  line L661 (3.8251, -17.4083) -> (3.907, -17.4302)
  line L662 (3.907, -17.4302) -> (3.9889, -17.4083)
  line L663 (3.9889, -17.4083) -> (4.0488, -17.3484)
  line L664 (-13.3262, 16.6651) -> (-13.3595, 16.674)
  line L665 (4.0488, -17.3484) -> (4.0563, -17.3203)
  line L666 (-13.3467, 16.7541) -> (-13.4072, 16.8146)
  line L667 (-13.633, 16.5888) -> (-13.579, 16.5229)
  line L668 (-13.633, 16.7541) -> (-13.6552, 16.6714)
  line L669 (-13.5013, 16.5922) -> (-13.522, 16.5147)
  line L670 (-13.6552, 16.6714) -> (-13.633, 16.5888)
  line L671 (-13.4072, 16.5282) -> (-13.3467, 16.5888)
  line L672 (-13.3467, 16.5888) -> (-13.3262, 16.6651)
  line L673 (1.8198, -17.435) -> (1.7976, -17.3523)
  line L674 (1.7976, -17.3523) -> (1.7371, -17.2918)
  line L675 (-13.4899, 16.5061) -> (-13.4072, 16.5282)
  line L676 (1.7371, -17.2918) -> (1.6544, -17.2697)
  line L677 (1.5112, -17.5177) -> (1.5717, -17.5782)
  line L678 (1.6544, -17.2697) -> (1.5717, -17.2918)
  line L679 (-13.3262, 16.6651) -> (-13.3467, 16.7541)
  line L680 (1.5717, -17.2918) -> (1.5112, -17.3523)
  line L681 (1.5112, -17.3523) -> (1.4891, -17.435)
  line L682 (1.4891, -17.435) -> (1.5112, -17.5177)
  line L683 (1.7371, -17.5782) -> (1.7976, -17.5177)
  line L684 (-13.4072, 16.8146) -> (-13.4899, 16.8368)
  line L685 (1.7976, -17.5177) -> (1.8198, -17.435)
  line L686 (-4.0565, -17.3523) -> (-4.117, -17.2918)
  line L687 (-4.117, -17.2918) -> (-4.1997, -17.2697)
  line L688 (-4.1997, -17.2697) -> (-4.2823, -17.2918)
  line L689 (-4.3429, -17.5177) -> (-4.2823, -17.5782)
  line L690 (-4.3429, -17.3523) -> (-4.365, -17.435)
  line L691 (-4.365, -17.435) -> (-4.3429, -17.5177)
  line L692 (-4.2823, -17.5782) -> (-4.1997, -17.6003)
  line L693 (5.0013, -14.3807) -> (4.9792, -14.298)
  line L694 (-4.1997, -17.6003) -> (-4.117, -17.5782)
  line L695 (-4.117, -17.5782) -> (-4.0565, -17.5177)
  line L696 (-4.0565, -17.5177) -> (-4.0343, -17.435)
  line L697 (-13.3467, -13.4072) -> (-13.4072, -13.3467)
  line L698 (-0.2705, -17.3523) -> (-0.2926, -17.435)
  line L699 (-0.2926, -17.435) -> (-0.2705, -17.5177)
  line L700 (-13.4007, 10.5628) -> (-13.3785, 10.4801)
  line L701 (-13.2711, 10.4607) -> (-13.2529, 10.3927)
  line L702 (-1.7658, -17.3523) -> (-1.8263, -17.2918)
  line L703 (-2.0323, -17.3484) -> (-1.9724, -17.4083)
  line L704 (-1.9724, -17.4083) -> (-1.8905, -17.4302)
  line L705 (-1.8905, -17.4302) -> (-1.8086, -17.4083)
  line L706 (-1.8086, -17.4083) -> (-1.7658, -17.3523)
  line L707 (-1.7436, -17.435) -> (-1.7658, -17.3523)
  line L708 (-13.3785, 10.6455) -> (-13.4007, 10.5628)
  line L709 (-13.2492, 10.5426) -> (-13.2711, 10.4607)
  line L710 (-1.8263, -17.2918) -> (-1.9089, -17.2697)
  line L711 (-1.9089, -17.2697) -> (-1.9916, -17.2918)
  line L712 (-13.1527, 10.4196) -> (-13.0921, 10.4801)
  line L713 (-13.5157, -13.3314) -> (-13.5232, -13.3595)
  line L714 (-2.0521, -17.3523) -> (-2.0743, -17.435)
  line L715 (-13.5232, -13.3595) -> (-13.5013, -13.4413)
  line L716 (-2.0743, -17.435) -> (-2.0521, -17.5177)
  line L717 (-13.5013, -13.4413) -> (-13.4413, -13.5013)
  line L718 (-2.0521, -17.5177) -> (-1.9916, -17.5782)
  line L719 (-13.318, 10.706) -> (-13.3785, 10.6455)
  line L720 (-13.1893, 10.6025) -> (-13.2492, 10.5426)
  line L721 (-1.9916, -17.5782) -> (-1.9089, -17.6003)
  line L722 (-13.3785, 10.4801) -> (-13.318, 10.4196)
  line L723 (-13.4413, -13.5013) -> (-13.3595, -13.5232)
  line L724 (-1.9089, -17.6003) -> (-1.8263, -17.5782)
  line L725 (-13.3595, -13.5232) -> (-13.3314, -13.5157)
  line L726 (-1.8263, -17.5782) -> (-1.7658, -17.5177)
  line L727 (-1.7658, -17.5177) -> (-1.7436, -17.435)
  line L728 (-1.2162, 5.8133) -> (-1.2761, 5.7533)
  line L729 (-8.5266, 13.4899) -> (-8.2721, 13.5581)
  line L730 (-1.2477, 16.3432) -> (-1.3045, 16.4)
  line L731 (-0.985, 5.7255) -> (-0.9925, 5.7533)
  line L732 (-9.1788, 17.5177) -> (-9.201, 17.435)
  line L733 (-12.9715, -16.6541) -> (-13.2927, -16.8879)
  line L734 (13.1972, 2.1635) -> (13.2194, 2.0808)
  line L735 (-17.1805, 13.0189) -> (-17.2631, 12.9967)
  line L736 (-17.025, 12.8902) -> (-17.0963, 12.8711)
  line L737 (-2.7552, 3.8338) -> (-2.8157, 3.7733)
  line L738 (-8.9675, 14.2534) -> (-9.0357, 13.9989)
  line L739 (-8.8808, 14.1157) -> (-8.9483, 13.8636)
  line L740 (-0.9925, 5.7533) -> (-1.0524, 5.8133)
  line L741 (-1.2761, 5.7533) -> (-1.298, 5.6715)
  line L742 (-9.0357, 13.9989) -> (-8.9675, 13.7444)
  line L743 (-8.9483, 13.8636) -> (-8.8977, 13.6746)
  line L744 (-17.3237, 12.9362) -> (-17.3458, 12.8535)
  line L745 (-17.1562, 12.8112) -> (-17.1782, 12.7293)
  line L746 (-1.2886, 5.8095) -> (-1.3107, 5.7268)
  line L747 (-1.3107, 5.7268) -> (-1.298, 5.6715)
  line L748 (14.6352, 2.5833) -> (14.5525, 2.5612)
  line L749 (-8.2721, 14.4398) -> (-8.5266, 14.508)
  line L750 (-8.1921, 14.3002) -> (-8.4442, 14.3677)
  line L751 (-1.0022, 5.8095) -> (-1.0627, 5.87)
  line L752 (-17.3458, 12.8535) -> (-17.3237, 12.7709)
  line L753 (-17.1782, 12.7293) -> (-17.168, 12.6915)
  line L754 (-0.9735, 3.5474) -> (-0.8908, 3.5253)
  line L755 (-8.5266, 14.508) -> (-8.7811, 14.4398)
  line L756 (-8.4442, 14.3677) -> (-8.6963, 14.3002)
  line L757 (18.4531, 14.3807) -> (18.4444, 14.647)
  line L758 (-17.3523, 9.4334) -> (-17.435, 9.4555)
  line L759 (18.4422, -13.6955) -> (18.4531, -13.3626)
  line L760 (18.2796, -14.6801) -> (18.3553, -14.3557)
  line L761 (18.3553, -14.3557) -> (18.4095, -14.027)
  line L762 (18.4095, -14.027) -> (18.4422, -13.6955)
  line L763 (18.0656, -15.3106) -> (18.1829, -14.9989)
  line L764 (18.1829, -14.9989) -> (18.2796, -14.6801)
  line L765 (-6.9534, -18.4531) -> (13.3626, -18.4531)
  line L766 (15.6141, -17.9281) -> (15.9078, -17.7711)
  line L767 (-16.7895, -15.1443) -> (-16.9259, -15.6533)
  line L768 (15.9078, -17.7711) -> (16.1907, -17.5952)
  line L769 (17.9281, -15.6141) -> (18.0656, -15.3106)
  line L770 (16.1907, -17.5952) -> (16.4615, -17.4012)
  line L771 (16.4615, -17.4012) -> (16.719, -17.1898)
  line L772 (16.719, -17.1898) -> (16.9621, -16.9621)
  line L773 (-8.953, 17.2918) -> (-8.8925, 17.3523)
  line L774 (-15.1443, 16.535) -> (-15.6533, 16.6714)
  line L775 (14.6801, -18.2796) -> (14.9989, -18.1829)
  line L776 (14.9989, -18.1829) -> (15.3106, -18.0656)
  line L777 (15.3106, -18.0656) -> (15.6141, -17.9281)
  line L778 (16.9621, -16.9621) -> (17.1898, -16.719)
  line L779 (17.1898, -16.719) -> (17.4012, -16.4615)
  line L780 (-4.2851, 13.0191) -> (-4.367, 12.9971)
  line L781 (17.5952, -16.1907) -> (17.7711, -15.9078)
  line L782 (-14.8897, -15.6533) -> (-15.0261, -15.1443)
  line L783 (17.7711, -15.9078) -> (17.9281, -15.6141)
  line L784 (14.2626, -3.4361) -> (14.6352, -3.8087)
  line L785 (13.3626, -18.4531) -> (13.6955, -18.4422)
  line L786 (-16.051, 13.1907) -> (-16.0732, 13.1081)
  line L787 (16.0062, -2.8988) -> (15.8711, -2.3946)
  line L788 (13.6955, -18.4422) -> (14.027, -18.4095)
  line L789 (14.027, -18.4095) -> (14.3557, -18.3553)
  line L790 (14.3557, -18.3553) -> (14.6801, -18.2796)
  line L791 (-2.8157, 3.6079) -> (-2.7885, 3.5731)
  line L792 (-2.8104, 3.6549) -> (-2.8157, 3.6079)
  line L793 (18.4531, -1.8628) -> (18.4531, 14.3807)
  line L794 (-12.4558, 13.0254) -> (-12.4337, 13.1081)
  line L795 (18.4444, 14.647) -> (18.4183, 14.9122)
  line L796 (18.4183, 14.9122) -> (18.3748, 15.1752)
  line L797 (-14.2694, 17.5177) -> (-14.2915, 17.435)
  line L798 (-14.1314, 17.3484) -> (-14.1508, 17.2762)
  line L799 (18.3748, 15.1752) -> (18.3143, 15.4347)
  line L800 (18.3143, 15.4347) -> (18.237, 15.6897)
  line L801 (18.237, 15.6897) -> (18.1431, 15.9391)
  line L802 (18.1431, 15.9391) -> (18.0331, 16.1819)
  line L803 (18.0331, 16.1819) -> (17.9075, 16.4169)
  line L804 (17.9075, 16.4169) -> (17.7668, 16.6432)
  line L805 (-4.367, 12.9971) -> (-4.4269, 12.9372)
  line L806 (17.7668, 16.6432) -> (17.6116, 16.8598)
  line L807 (17.6116, 16.8598) -> (17.4425, 17.0658)
  line L808 (17.4425, 17.0658) -> (17.2603, 17.2603)
  line L809 (17.2603, 17.2603) -> (17.0658, 17.4425)
  line L810 (17.0658, 17.4425) -> (16.8598, 17.6116)
  line L811 (16.8598, 17.6116) -> (16.6432, 17.7668)
  line L812 (16.6432, 17.7668) -> (16.4169, 17.9075)
  line L813 (16.4169, 17.9075) -> (16.1819, 18.0331)
  line L814 (16.1819, 18.0331) -> (15.9391, 18.1431)
  line L815 (15.9391, 18.1431) -> (15.6897, 18.237)
  line L816 (15.6897, 18.237) -> (15.4347, 18.3143)
  line L817 (15.4347, 18.3143) -> (15.1752, 18.3749)
  line L818 (15.1752, 18.3749) -> (14.9122, 18.4183)
  line L819 (14.9122, 18.4183) -> (14.647, 18.4444)
  line L820 (16.1624, -2.927) -> (16.026, -2.418)
  line L821 (14.647, 18.4444) -> (14.3807, 18.4531)
  line L822 (14.3807, 18.4531) -> (-1.6083, 18.4531)
  line L823 (-8.1218, 18.4531) -> (-13.3626, 18.4531)
  line L824 (-13.3626, 18.4531) -> (-13.6955, 18.4422)
  line L825 (11.4696, 12.7709) -> (11.4917, 12.8535)
  line L826 (-15.2556, -0.719) -> (-15.2335, -0.6363)
  line L827 (-13.6955, 18.4422) -> (-14.027, 18.4096)
  line L828 (16.9261, 7.0578) -> (16.9042, 7.1397)
  line L829 (-14.027, 18.4096) -> (-14.3557, 18.3553)
  line L830 (-14.3557, 18.3553) -> (-14.6801, 18.2796)
  line L831 (-14.6801, 18.2796) -> (-14.9989, 18.1829)
  line L832 (-14.9989, 18.1829) -> (-15.3106, 18.0656)
  line L833 (-15.3106, 18.0656) -> (-15.6141, 17.9281)
  line L834 (-15.6141, 17.9281) -> (-15.9078, 17.7711)
  line L835 (5.4723, 16.535) -> (4.9632, 16.6714)
  line L836 (-15.9078, 17.7711) -> (-16.1907, 17.5952)
  line L837 (-16.1907, 17.5952) -> (-16.4615, 17.4012)
  line L838 (-16.4615, 17.4012) -> (-16.719, 17.1898)
  line L839 (-16.719, 17.1898) -> (-16.9621, 16.9621)
  line L840 (-16.9621, 16.9621) -> (-17.1898, 16.719)
  line L841 (-17.1898, 16.719) -> (-17.4012, 16.4615)
  line L842 (-17.4012, 16.4615) -> (-17.5952, 16.1907)
  line L843 (-17.5952, 16.1907) -> (-17.7711, 15.9078)
  line L844 (-17.7711, 15.9078) -> (-17.9281, 15.6141)
  line L845 (-17.9281, 15.6141) -> (-18.0656, 15.3106)
  line L846 (-18.0656, 15.3106) -> (-18.1829, 14.9989)
  line L847 (-18.1829, 14.9989) -> (-18.2796, 14.6801)
  line L848 (-18.2796, 14.6801) -> (-18.3553, 14.3557)
  line L849 (-18.3553, 14.3557) -> (-18.4095, 14.027)
  line L850 (-18.4095, 14.027) -> (-18.4422, 13.6955)
  line L851 (-18.4422, 13.6955) -> (-18.4531, 13.3626)
  line L852 (-1.2886, 5.6442) -> (-1.228, 5.5836)
  line L853 (-16.4089, -14.7796) -> (-16.6273, -14.9979)
  line L854 (-12.0008, 17.435) -> (-11.9786, 17.3523)
  line L855 (-11.7528, 17.5782) -> (-11.8354, 17.6003)
  line L856 (-6.9534, -18.4531) -> (-7.1287, -18.0967)
  line L857 (-11.9786, 17.3523) -> (-11.9181, 17.2918)
  line L858 (-7.1287, -18.0967) -> (-7.3378, -17.7589)
  line L859 (14.6352, 2.2527) -> (14.7179, 2.2748)
  line L860 (-7.3378, -17.7589) -> (-7.5785, -17.4429)
  line L861 (-7.5785, -17.4429) -> (-7.8486, -17.1517)
  line L862 (-7.8486, -17.1517) -> (-8.1456, -16.8879)
  line L863 (-8.1456, -16.8879) -> (-8.4667, -16.6541)
  line L864 (-8.4667, -16.6541) -> (-8.8089, -16.4524)
  line L865 (-8.8089, -16.4524) -> (-9.1691, -16.2848)
  line L866 (-9.1691, -16.2848) -> (-9.5437, -16.1527)
  line L867 (-9.201, 17.435) -> (-9.1788, 17.3523)
  line L868 (-9.5437, -16.1527) -> (-9.9293, -16.0575)
  line L869 (-9.9293, -16.0575) -> (-10.3224, -16)
  line L870 (-10.3224, -16) -> (-10.7191, -15.9808)
  line L871 (-10.7191, -15.9808) -> (-11.1159, -16)
  line L872 (-11.1159, -16) -> (-11.5089, -16.0575)
  line L873 (-11.5089, -16.0575) -> (-11.8946, -16.1527)
  line L874 (-11.8946, -16.1527) -> (-12.2692, -16.2848)
  line L875 (-12.2692, -16.2848) -> (-12.6293, -16.4524)
  line L876 (-12.6293, -16.4524) -> (-12.9715, -16.6541)
  line L877 (-13.2927, -16.8879) -> (-13.5897, -17.1517)
  line L878 (18.4531, -1.8628) -> (18.1449, -2.0145)
  line L879 (-15.9905, 13.2513) -> (-16.051, 13.1907)
  line L880 (-15.0261, -15.1443) -> (-15.3988, -14.7716)
  line L881 (18.1449, -2.0145) -> (17.8528, -2.1953)
  line L882 (17.8528, -2.1953) -> (17.5795, -2.4035)
  line L883 (-15.1443, 14.7716) -> (-14.7716, 15.1443)
  line L884 (17.5795, -2.4035) -> (17.3276, -2.6371)
  line L885 (17.3276, -2.6371) -> (17.0995, -2.8939)
  line L886 (17.0913, 7.1267) -> (17.0691, 7.2094)
  line L887 (17.0995, -2.8939) -> (16.8973, -3.1716)
  line L888 (16.8973, -3.1716) -> (16.7229, -3.4676)
  line L889 (16.7229, -3.4676) -> (16.5779, -3.779)
  line L890 (16.5779, -3.779) -> (16.4637, -4.103)
  line L891 (16.4637, -4.103) -> (16.3813, -4.4365)
  line L892 (16.3813, -4.4365) -> (16.3316, -4.7764)
  line L893 (16.3316, -4.7764) -> (16.315, -5.1196)
  line L894 (16.315, -5.1196) -> (16.3316, -5.4627)
  line L895 (16.3316, -5.4627) -> (16.3813, -5.8026)
  line L896 (16.3813, -5.8026) -> (16.4637, -6.1361)
  line L897 (-8.8925, 17.5177) -> (-8.953, 17.5782)
  line L898 (16.4637, -6.1361) -> (16.5779, -6.4601)
  line L899 (16.5779, -6.4601) -> (16.7229, -6.7715)
  line L900 (16.7229, -6.7715) -> (16.8973, -7.0675)
  line L901 (-11.6701, 17.435) -> (-11.6922, 17.5177)
  line L902 (16.8973, -7.0675) -> (17.0995, -7.3452)
  line L903 (17.0995, -7.3452) -> (17.3276, -7.6021)
  line L904 (17.3276, -7.6021) -> (17.5795, -7.8357)
  line L905 (10.6455, 13.5058) -> (10.5628, 13.5279)
  line L906 (17.5795, -7.8357) -> (17.8528, -8.0438)
  line L907 (10.6245, 13.2334) -> (10.6025, 13.3153)
  line L908 (17.8528, -8.0438) -> (18.1449, -8.2246)
  line L909 (-14.7716, 15.1443) -> (-14.6352, 15.6533)
  line L910 (-7.9701, 18.1449) -> (-7.7893, 17.8528)
  line L911 (-7.7893, 17.8528) -> (-7.5812, 17.5795)
  line L912 (-15.6533, 14.6352) -> (-15.1443, 14.7716)
  line L913 (-7.5812, 17.5795) -> (-7.3475, 17.3276)
  line L914 (-7.3475, 17.3276) -> (-7.0907, 17.0995)
  line L915 (-7.0907, 17.0995) -> (-6.813, 16.8973)
  line L916 (-6.813, 16.8973) -> (-6.517, 16.7229)
  line L917 (-6.517, 16.7229) -> (-6.2056, 16.5779)
  line L918 (-14.1262, 17.6003) -> (-14.2088, 17.5782)
  line L919 (-13.9896, 17.4302) -> (-14.0715, 17.4083)
  line L920 (-6.2056, 16.5779) -> (-5.8816, 16.4637)
  line L921 (-5.8816, 16.4637) -> (-5.5481, 16.3813)
  line L922 (-5.5481, 16.3813) -> (-5.2082, 16.3316)
  line L923 (-5.2082, 16.3316) -> (-4.865, 16.315)
  line L924 (-4.865, 16.315) -> (-4.5219, 16.3316)
  line L925 (-4.5219, 16.3316) -> (-4.182, 16.3813)
  line L926 (14.6352, -15.6533) -> (14.7716, -16.1624)
  line L927 (-4.182, 16.3813) -> (-3.8485, 16.4637)
  line L928 (-3.8485, 16.4637) -> (-3.5245, 16.5779)
  line L929 (-15.25, -16.3752) -> (-15.0316, -16.1569)
  line L930 (-3.5245, 16.5779) -> (-3.2131, 16.7229)
  line L931 (-3.2131, 16.7229) -> (-2.9171, 16.8973)
  line L932 (-2.9171, 16.8973) -> (-2.6394, 17.0995)
  line L933 (-2.6394, 17.0995) -> (-2.3825, 17.3276)